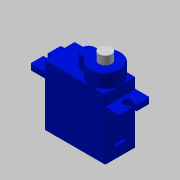
# Autodesk Inventor part: Servo Motor SG90
Saved by Autodesk Inventor 2019.2 (Build 232265000, 265)
## iProperties
Created: 2018-01-08
Part Number: Servo Motor SG90
Material: Generisch
Document SubType Name: Modeling
Designer: user
Density: 4 g/cm^3
Appearance: Stein - Blau
Mass: 24.3384 g
Surface Area: 24.0512 cm^2
Volume: 6.08459 cm^3
Author: user
Autodesk Inventor part; units mm, degrees
ref_plane "YZ Plane" through (0, 0, 0) normal (1, 0, 0) x (0, 1, 0)
ref_plane "XZ Plane" through (0, 0, 0) normal (0, 1, 0) x (-1, 0, 0)
sketch "스케치1" plane through (0, 0, 0) normal (0, 0, 1) x (1, 0, 0)
  line L0 (-11, -5.5) -> (11, -5.5)
  line L1 (11, -5.5) -> (11, 5.5)
  line L2 (11, 5.5) -> (-11, 5.5)
  line L3 (-11, 5.5) -> (-11, -5.5)
  line L4 (-11, -5.5) -> (11, 5.5) construction
  line L5 (11, -5.5) -> (-11, 5.5) construction
  point P0 (0, 0)
  dimension "d0" = 22
  dimension "d1" = 11
  constraints: 12 end point, 2 midpoint, 2 parallel, 1 horizontal, 1 perpendicular
  measures "d0" distance of L2.end L1.end
  measures "d1" distance of L1.end L0.end
extrude "돌출1" add sketch "스케치1" along normal blind 22
ref_plane "작업 평면1" through (0, 0, 16) normal (0, 0, -1) x (-1, 0, 0)
sketch "스케치2" plane through (0, 0, 16) normal (0, 0, -1) x (-1, 0, 0)
  line L0 (16, -5.5) -> (-16, -5.5)
  line L1 (-16, 5.5) -> (16, 5.5)
  line L2 (16, 5.5) -> (16, 0.75)
  line L3 (-11, -5.5) -> (-11, 5.5)
  line L4 (11, 5.5) -> (11, -5.5)
  line L5 (11, -5.5) -> (-11, -5.5)
  line L6 (0, -5.5) -> (0, 5.5) construction
  arc A0 (14.799038, -0.75) -> (14.799038, 0.75) centre (13.5, 0) ccw construction
  line L7 (-11, 5.5) -> (11, 5.5)
  line L8 (16, -0.75) -> (14.799038, -0.75)
  line L9 (16, 0.75) -> (14.799038, 0.75)
  line L10 (13.5, 0) -> (0, 0) construction
  line L11 (16, -0.75) -> (16, -5.5)
  line L12 (16, 0.75) -> (16, -0.75) construction
  arc A1 (12, 0) -> (14.799038, -0.75) centre (13.5, 0) ccw
  arc A2 (14.799038, 0.75) -> (12, 0) centre (13.5, 0) ccw
  line L13 (-16, -0.75) -> (-14.799038, -0.75)
  line L14 (-16, 0.75) -> (-14.799038, 0.75)
  arc A3 (-14.799038, -0.75) -> (-12, 0) centre (-13.5, 0) ccw
  arc A4 (-12, 0) -> (-14.799038, 0.75) centre (-13.5, 0) ccw
  line L15 (-16, -5.5) -> (-16, -0.75)
  line L16 (-16, 0.75) -> (-16, 5.5)
  point P0 (0, 0)
  dimension "d6" = 5
  dimension "d7" = 3
  dimension "d8" = 2.5
  dimension "d9" = 1.5
  constraints: 26 end point, 10 point on circle, 7 parallel, 6 symmetric about line, 5 centre point, 5 perpendicular, 3 midpoint, 2 collinear, 2 horizontal, 1 horizontal alignment, 1 point on line, 3 other
  measures "d6" distance between parallel lines of L4 L2
  measures "d7" diameter of A0
  measures "d8" distance from line of L2 L10.start
  measures "d9" distance between parallel lines of L9 L8
extrude "돌출2" add sketch "스케치2" against normal blind 2 contours L0 L4 L1 L2 L9 A2 A1 L8 L11 | L0 L15 L13 A3 A4 L14 L16 L1 L3
sketch "스케치3" plane through (0, 0, 22) normal (0, 0, 1) x (1, 0, 0)
  line L0 (-11, -5.5) -> (11, -5.5)
  line L1 (11, -5.5) -> (11, 5.5)
  line L2 (11, 5.5) -> (-11, 5.5)
  arc A0 (0.601021, -2.5) -> (0.601021, 2.5) centre (5.5, 0) ccw
  line L3 (5.5, 0) -> (-0.5, 0) construction
  line L4 (0.601021, 2.5) -> (-0.5, 2.5)
  line L5 (-0.5, -2.5) -> (0.601021, -2.5)
  arc A1 (-0.5, 2.5) -> (-0.5, -2.5) centre (-0.5, 0) ccw
  point P0 (0, 0)
  point P1 (2.5, 0)
  dimension "d12" = 6
  dimension "d13" = 5
  constraints: 8 end point, 5 tangent, 4 point on circle, 3 horizontal, 2 centre point, 1 midpoint, 1 parallel
  measures "d12" distance of L3.start L3.end
  measures "d13" diameter of A1
extrude "돌출3" add sketch "스케치3" along normal blind 5 contours A0 L5 A1 L4
fillet "모깎기1" radius 0.5 23 edges at (16, -5.5, 17) (16, 5.5, 17) (11, -5.5, 20) (11, 5.5, 20) (11, -5.5, 8) (11, -2.75, 22) (11, 2.75, 22) (11, 0, 27) (-3, 0, 27) (0.0505, 2.5, 27) (0.0505, -2.5, 27) (-2.75, -5.5, 22) (8.25, -5.5, 22) (-11, 0, 22) (-2.75, 5.5, 22) (8.25, 5.5, 22) (-16, -5.5, 17) (-16, 5.5, 17) (-11, -5.5, 8) (-11, -5.5, 20) (-11, 5.5, 20) (-11, 5.5, 8) (11, 5.5, 8)
sketch "스케치4" plane through (0, 0, 27) normal (0, 0, 1) x (1, 0, 0)
  arc A0 (0.917424, -2) -> (0.917424, 2) centre (5.5, 0) ccw
  circle A1 centre (5.5, 0) radius 2.25
  point P0 (0, 0)
  dimension "d17" = 4.5
  constraints: 1 centre point, 1 coincident
  measures "d17" diameter of A1
extrude "돌출4" add sketch "스케치4" along normal blind 3
sketch "스케치6" plane through (11, -5, 0) normal (1, 0, 0) x (0, 0, -1)
  line L0 (0, 0) -> (0, 10) projected
  line L1 (-3.8, 3.2) -> (-5, 3.2)
  line L2 (-5, 3.2) -> (-5, 6.8)
  line L3 (-5, 6.8) -> (-3.8, 6.8)
  line L4 (-3.8, 6.8) -> (-3.8, 3.2)
  line L5 (-3.8, 3.2) -> (-5, 6.8) construction
  line L6 (-5, 3.2) -> (-3.8, 6.8) construction
  line L7 (-4.4, 5) -> (0, 5) construction
  dimension "d25" = 1.2
  dimension "d26" = 3.6
  dimension "d27" = 5
  constraints: 14 end point, 2 midpoint, 2 parallel, 2 perpendicular, 1 horizontal
  measures "d25" distance of L2.end L3.end
  measures "d26" distance of L1.end L2.end
  measures "d27" distance between parallel lines of L0 L2
extrude "돌출6" cut sketch "스케치6" against normal blind 1
